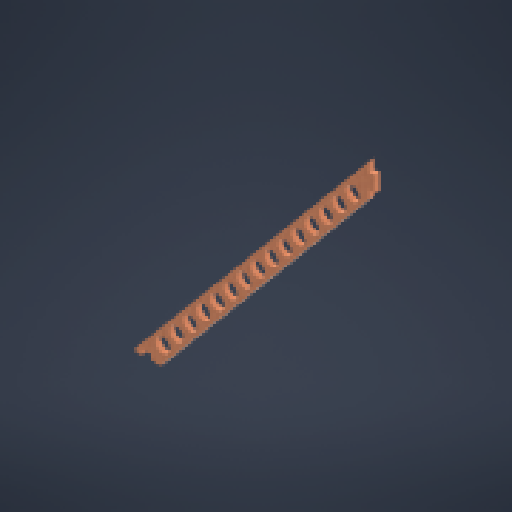
# Autodesk Inventor part: SUPPORTS_TREBUCHET
Saved by Autodesk Inventor 2026.2 (Build 302298010, 298A)
## iProperties
Created: 2026-02-18
Part Number: SUPPORTS_TREBUCHET
Material: Wood (Oak)
Document SubType Name: Modeling
Designer: 4aida
Density: 0.76 g/cm^3
Appearance: White Oak - Natural Medium Gloss
Mass: 120.158 g
Surface Area: 578.245 cm^2
Volume: 158.102 cm^3
Author: 4aida
Autodesk Inventor part; units mm, degrees
ref_plane "YZ Plane" through (0, 0, 0) normal (1, 0, 0) x (0, 1, 0)
ref_plane "XZ Plane" through (0, 0, 0) normal (0, 1, 0) x (-1, 0, 0)
ref_plane "XY Plane" through (0, 0, 0) normal (0, 0, 1) x (1, 0, 0)
sketch "Sketch1" plane through (0, 0, 0) normal (0, 0, 1) x (1, 0, 0)
  line L0 (201.8785, 270.226) -> (-226.7465, -240.5894)
  line L1 (-226.7465, -240.5894) -> (-177.0105, -240.5894)
  line L2 (-177.0105, -240.5894) -> (201.8785, 210.9529)
  line L3 (201.8785, 210.9529) -> (201.8785, 270.226)
  line L4 (-12.434, 14.8183) -> (12.434, -14.8183) construction
  point P0 (0, 0)
  point P1 (0, 0)
  dimension "d0" = 50
  dimension "d1" = 38.1
  dimension "d2" = 428.625
  constraints: 10 end point, 3 midpoint, 1 coincident, 1 horizontal, 1 parallel, 1 perpendicular
  measures "d0" angle of L1 L2
  measures "d1" distance between parallel lines of L0 L2
  measures "d2" distance from line of L3 L0.end
extrude "Extrusion1" add sketch "Sketch1" along normal blind 9.525
sketch "Sketch2" plane through (0, 0, 9.525) normal (0, 0, 1) x (1, 0, 0)
  line L0 (201.8785, 210.9529) -> (201.8785, 270.226) projected
  line L1 (201.8785, 225.9981) -> (211.4035, 224.4106)
  line L2 (211.4035, 224.4106) -> (211.4035, 254.4106)
  line L3 (211.4035, 254.4106) -> (201.8785, 252.8231)
  line L4 (-226.7465, -240.5894) -> (-177.0105, -240.5894) projected
  point P0 (0, 0)
  point P1 (211.4035, 239.4106)
  dimension "d5" = 480
  dimension "d6" = 9.525
  dimension "d8" = 1.5875
  dimension "d9" = 30
  constraints: 6 end point, 2 point on line, 1 equal length, 1 midpoint, 1 parallel
  measures "d5" distance from line of L4 point (211.403, 239.411)
  measures "d6" distance between parallel lines of L0 L2
  measures "d8" vertical distance of L2.end L3.end
  measures "d9" distance of L1.end L2.end
extrude "Extrusion2" add sketch "Sketch2" against normal up to surface (9.525 mm away)
sketch "Sketch3" plane through (0, 0, 9.525) normal (0, 0, 1) x (1, 0, 0)
  circle A0 centre (0, 0) radius 12.7
  line L0 (201.8785, 270.226) -> (-226.7465, -240.5894) projected
  circle A1 centre (-24.4902, -29.1863) radius 12.7
  circle A2 centre (-48.9804, -58.3726) radius 12.7
  circle A3 centre (-73.4706, -87.5589) radius 12.7
  circle A4 centre (-97.9608, -116.7452) radius 12.7
  circle A5 centre (-122.451, -145.9315) radius 12.7
  circle A6 centre (-146.9412, -175.1178) radius 12.7
  circle A7 centre (-171.4315, -204.3041) radius 12.7
  circle A8 centre (24.4902, 29.1863) radius 12.7
  circle A9 centre (0, 0) radius 12.7
  circle A10 centre (-24.4902, -29.1863) radius 12.7
  circle A11 centre (-48.9804, -58.3726) radius 12.7
  circle A12 centre (-73.4706, -87.5589) radius 12.7
  circle A13 centre (-97.9608, -116.7452) radius 12.7
  circle A14 centre (-122.451, -145.9315) radius 12.7
  circle A15 centre (-146.9412, -175.1178) radius 12.7
  circle A16 centre (48.9804, 58.3726) radius 12.7
  circle A17 centre (24.4902, 29.1863) radius 12.7
  circle A18 centre (0, 0) radius 12.7
  circle A19 centre (-24.4902, -29.1863) radius 12.7
  circle A20 centre (-48.9804, -58.3726) radius 12.7
  circle A21 centre (-73.4706, -87.5589) radius 12.7
  circle A22 centre (-97.9608, -116.7452) radius 12.7
  circle A23 centre (-122.451, -145.9315) radius 12.7
  circle A24 centre (73.4706, 87.5589) radius 12.7
  circle A25 centre (48.9804, 58.3726) radius 12.7
  circle A26 centre (24.4902, 29.1863) radius 12.7
  circle A27 centre (0, 0) radius 12.7
  circle A28 centre (-24.4902, -29.1863) radius 12.7
  circle A29 centre (-48.9804, -58.3726) radius 12.7
  circle A30 centre (-73.4706, -87.5589) radius 12.7
  circle A31 centre (-97.9608, -116.7452) radius 12.7
  circle A32 centre (97.9608, 116.7452) radius 12.7
  circle A33 centre (73.4706, 87.5589) radius 12.7
  circle A34 centre (48.9804, 58.3726) radius 12.7
  circle A35 centre (24.4902, 29.1863) radius 12.7
  circle A36 centre (0, 0) radius 12.7
  circle A37 centre (-24.4902, -29.1863) radius 12.7
  circle A38 centre (-48.9804, -58.3726) radius 12.7
  circle A39 centre (-73.4706, -87.5589) radius 12.7
  circle A40 centre (122.451, 145.9315) radius 12.7
  circle A41 centre (97.9608, 116.7452) radius 12.7
  circle A42 centre (73.4706, 87.5589) radius 12.7
  circle A43 centre (48.9804, 58.3726) radius 12.7
  circle A44 centre (24.4902, 29.1863) radius 12.7
  circle A45 centre (0, 0) radius 12.7
  circle A46 centre (-24.4902, -29.1863) radius 12.7
  circle A47 centre (-48.9804, -58.3726) radius 12.7
  circle A48 centre (146.9412, 175.1178) radius 12.7
  circle A49 centre (122.451, 145.9315) radius 12.7
  circle A50 centre (97.9608, 116.7452) radius 12.7
  circle A51 centre (73.4706, 87.5589) radius 12.7
  circle A52 centre (48.9804, 58.3726) radius 12.7
  circle A53 centre (24.4902, 29.1863) radius 12.7
  circle A54 centre (0, 0) radius 12.7
  circle A55 centre (-24.4902, -29.1863) radius 12.7
  circle A56 centre (171.4315, 204.3041) radius 12.7
  circle A57 centre (146.9412, 175.1178) radius 12.7
  circle A58 centre (122.451, 145.9315) radius 12.7
  circle A59 centre (97.9608, 116.7452) radius 12.7
  circle A60 centre (73.4706, 87.5589) radius 12.7
  circle A61 centre (48.9804, 58.3726) radius 12.7
  circle A62 centre (24.4902, 29.1863) radius 12.7
  circle A63 centre (0, 0) radius 12.7
  dimension "d12" = 25.4
  dimension "d15" = 38.1
  dimension "d18" = 38.1
  constraints: 64 centre point, 1 coincident, 128 other
  measures "d12" diameter of A0
  measures "d15" distance of A0.centre A1.centre
  measures "d18" distance of A0.centre A8.centre
extrude "Extrusion3" cut sketch "Sketch3" against normal through all
chamfer "Chamfer1" distance 9.525 angle 11.388 1 edges at (-201.8785, -240.5894, 9.525) measured on face at (-201.8785, -240.5894, 9.025)
sketch "Sketch4" plane through (-226.7465, -240.5894, 0) normal (0, -0.9803126, 0.197452) x (1, 0, 0)
  line L0 (33.5993, 0) -> (16.1368, 0)
  line L1 (16.1368, 0) -> (16.1368, 17.2439)
  line L2 (16.1368, 17.2439) -> (33.5993, 17.2439)
  line L3 (33.5993, 17.2439) -> (33.5993, 0)
  line L4 (51.3458, 9.7163) -> (1.6098, 9.7163) projected
  line L5 (51.3458, 9.7163) -> (428.625, 98.4954) projected
  line L6 (428.625, 98.4954) -> (428.625, 101.4661) projected
  line L7 (428.625, 101.4661) -> (438.15, 101.1527) projected
  line L8 (438.15, 101.1527) -> (438.15, 107.0762) projected
  line L9 (438.15, 107.0762) -> (428.625, 106.7628) projected
  line L10 (428.625, 106.7628) -> (428.625, 110.199) projected
  line L11 (428.625, 110.199) -> (1.6098, 9.7163) projected
  ellipse E0 centre (202.2563, 51.0795) end of major axis (214.9563, 51.0795) minor radius 2.5076 projected
  ellipse E1 centre (128.7857, 33.7908) end of major axis (141.4857, 33.7908) minor radius 2.5076 projected
  ellipse E2 centre (55.315, 16.5021) end of major axis (68.015, 16.5021) minor radius 2.5076 projected
  ellipse E3 centre (79.8053, 22.265) end of major axis (92.5053, 22.265) minor radius 2.5076 projected
  ellipse E4 centre (373.6878, 91.4197) end of major axis (386.3878, 91.4197) minor radius 2.5076 projected
  ellipse E5 centre (251.2367, 62.6052) end of major axis (263.9367, 62.6052) minor radius 2.5076 projected
  ellipse E6 centre (300.2171, 74.131) end of major axis (312.9171, 74.131) minor radius 2.5076 projected
  ellipse E7 centre (177.7661, 45.3166) end of major axis (190.4661, 45.3166) minor radius 2.5076 projected
  ellipse E8 centre (153.2759, 39.5537) end of major axis (165.9759, 39.5537) minor radius 2.5076 projected
  ellipse E9 centre (275.7269, 68.3681) end of major axis (288.4269, 68.3681) minor radius 2.5076 projected
  ellipse E10 centre (324.7073, 79.8939) end of major axis (337.4073, 79.8939) minor radius 2.5076 projected
  ellipse E11 centre (226.7465, 56.8423) end of major axis (239.4465, 56.8423) minor radius 2.5076 projected
  ellipse E12 centre (398.178, 97.1826) end of major axis (410.878, 97.1826) minor radius 2.5076 projected
  ellipse E13 centre (104.2955, 28.0279) end of major axis (116.9955, 28.0279) minor radius 2.5076 projected
  ellipse E14 centre (349.1975, 85.6568) end of major axis (361.8975, 85.6568) minor radius 2.5076 projected
  line L12 (0, 0) -> (49.736, 0) projected
  point P0 (226.7465, 47.5049)
  point P1 (24.868, 0)
  point P2 (16.1368, 13.1347)
  dimension "d26" = 17.4625
  constraints: 8 end point, 2 midpoint, 2 parallel, 1 horizontal, 1 perpendicular, 1 point on line
  measures "d26" distance of L1.end L2.end
extrude "Extrusion4" cut sketch "Sketch4" against normal blind 9.525 contours L0 L1 L4 L3 | L4 L1 L11 L3
equation "\"d8\" = 0.166667 * d6"
body "Solid1"
